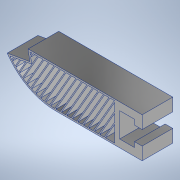
# Autodesk Inventor part: Finray_9_Kerbe_10deg_30deg20inf_PLA
Saved by Autodesk Inventor 2022 (Build 260153000, 153)
## iProperties
Created: 2022-02-28
Part Number: Finray_9_Kerbe_10deg_30deg20inf_PLA
Material: Generic
Document SubType Name: Modeling
Designer: richa
Density: 1 g/cm^3
Appearance: Aluminum - Flat
Author: richa
Autodesk Inventor part; units mm, degrees
ref_plane "YZ Plane" through (0, 0, 0) normal (1, 0, 0) x (0, 1, 0)
ref_plane "XZ Plane" through (0, 0, 0) normal (0, 1, 0) x (-1, 0, 0)
ref_plane "XY Plane" through (0, 0, 0) normal (0, 0, 1) x (1, 0, 0)
sketch "Sketch5" plane through (0, 0, 0) normal (0, 0, 1) x (1, 0, 0)
  line L0 (52.8, -15.6) -> (52.8, -10.6)
  line L1 (52.8, -10.6) -> (49.8, -10.6)
  line L2 (49.8, -10.6) -> (49.8, -12.6)
  line L3 (44, -12.6) -> (44, -3)
  line L4 (49.8, -3) -> (49.8, -5)
  line L5 (49.8, -5) -> (52.8, -5)
  line L6 (52.8, -5) -> (52.8, 0)
  line L7 (52.8, 0) -> (7.8, 0)
  line L8 (44, -3) -> (49.8, -3)
  line L9 (44, -12.6) -> (49.8, -12.6)
  line L10 (52.8, -15.6) -> (7.8, -15.6)
  line L11 (7.8, -15.6) -> (0, -15.6)
  line L12 (0, -15.6) -> (0, 0)
  line L13 (0, 0) -> (7.8, 0)
  point P0 (7.8, 0)
  dimension "d41" = 5.8
  dimension "d48" = 44
  dimension "d50" = 3
  dimension "d63" = 45
  dimension "d71" = 0
  dimension "d87" = 5.6
  dimension "d88" = 9.6
  dimension "d97" = 15.6
  constraints: 28 end point, 8 perpendicular, 4 collinear, 3 parallel, 2 horizontal, 1 vertical
  measures "d41" distance between parallel lines of L2 L3
  measures "d48" distance from line of L3 L12.end
  measures "d50" distance of L4.end L5.end
  measures "d63" distance of L0.start L10.end
  measures "d71" distance from line of L12.end L7
  measures "d87" distance from line of L0.end L5
  measures "d88" distance of L3.start L3.end
  measures "d97" distance of L11.end L12.end
extrude "Extrusion2" add sketch "Sketch5" along normal blind 12
sketch "Sketch8" plane through (0, 0, 0) normal (0, 0, -1) x (-1, 0, 0)
  line L0 (-8.1687, 0) -> (-8.8633, -3.9392)
  line L1 (-7.8, 0) -> (-1.143, 0) construction
  line L2 (0, -5.5021) -> (-8.8633, -3.9392)
  line L3 (-7.8, 0) -> (-8.1687, 0)
  line L4 (0, 0) -> (0, -15.6) projected
  line L5 (-52.8, 0) -> (0, 0) projected
  line L6 (-7.8, 0) -> (0, 0)
  line L7 (0, 0) -> (0, -5.5021)
  dimension "d80" = 100
  dimension "d95" = 4
  dimension "d96" = 9
  constraints: 12 end point, 2 collinear, 2 perpendicular, 1 horizontal, 1 point on line
  measures "d80" angle of L0 L1
  measures "d95" distance of L0.start L0.end
  measures "d96" distance of L2.start L0.end
extrude "Extrusion5" cut sketch "Sketch8" against normal through all
fillet "Fillet2" radius 23 1 edges at (0, -15.6, 6)
shell "Shell1" thickness 0.62 removed faces 1 at (23.9679, -7.5131, 12)
sketch "Sketch13" plane through (0, 0, 12) normal (0, 0, 1) x (1, 0, 0)
  line L0 (19.0404, -15.6) -> (52.8, -15.6) projected
  line L1 (42.0526, -15.6) -> (42.0526, 0)
  line L2 (52.8, 0) -> (8.1687, 0) projected
  line L3 (52.8, 0) -> (8.1687, 0) projected
  line L4 (52.8, -5) -> (52.8, 0) projected
  line L5 (49.8, -5) -> (52.8, -5) projected
  line L6 (49.8, -3) -> (49.8, -5) projected
  line L7 (44, -3) -> (49.8, -3) projected
  line L8 (44, -12.6) -> (44, -3) projected
  line L9 (49.8, -12.6) -> (44, -12.6) projected
  line L10 (49.8, -10.6) -> (49.8, -12.6) projected
  line L11 (52.8, -10.6) -> (49.8, -10.6) projected
  line L12 (52.8, -15.6) -> (52.8, -10.6) projected
  line L13 (42.0526, 0) -> (52.8, 0)
  line L14 (52.8, -5) -> (52.8, 0) projected
  line L15 (52.8, -5) -> (52.8, 0)
  line L16 (52.8, 0) -> (52.8, -5)
  line L17 (44, -12.6) -> (44, -3) projected
  line L18 (44, -3) -> (44, -12.6)
  line L19 (49.8, -12.6) -> (44, -12.6) projected
  line L20 (44, -12.6) -> (49.8, -12.6)
  line L21 (43.38, -13.22) -> (50.42, -13.22) projected
  line L22 (52.8, -10.6) -> (52.8, -15.6)
  line L23 (52.8, -15.6) -> (42.0526, -15.6)
  line L24 (44, -3) -> (49.8, -3) projected
  line L25 (44, -3) -> (49.8, -3)
  line L26 (49.8, -3) -> (49.8, -5)
  line L27 (49.8, -5) -> (52.8, -5)
  line L28 (52.8, -10.6) -> (49.8, -10.6)
  line L29 (49.8, -10.6) -> (49.8, -12.6)
  point P0 (0, 0)
  dimension "d102" = 10.7474
  constraints: 26 end point, 10 collinear, 2 point on line, 2 vertical, 1 parallel
  measures "d102" distance between parallel lines of L4 L1
extrude "Extrusion7" add sketch "Sketch13" against normal blind 12
sketch "Sketch14" plane through (8.9076, -0.62, 0.62) normal (0, 0, 1) x (1, 0, 0)
  line L0 (33.145, -14.36) -> (33.145, 0) projected
  line L1 (33.145, 0) -> (0, 0) projected
  line L2 (0.6739, -3.8221) -> (0, 0) projected
  line L3 (-7.835, -5.3225) -> (0.6739, -3.8221) projected
  arc A0 (-7.835, -5.3225) -> (10.1328, -14.36) centre (10.1328, 8.02) ccw projected
  line L4 (10.1328, -14.36) -> (33.145, -14.36) projected
  point P0 (-8.9076, 0.62)
extrude "Extrusion8" cut sketch "Sketch14" against normal blind 12
sketch "Sketch15" plane through (0, 0, 12) normal (0, 0, 1) x (1, 0, 0)
  line L0 (42.0526, -0.62) -> (8.9076, -0.62) construction
  line L1 (19.0404, -14.98) -> (42.0526, -14.98) projected
  line L2 (46.3521, -0.43) -> (46.6811, -0.62)
  line L3 (46.6811, -0.62) -> (38.2807, -15.17)
  line L4 (38.2807, -15.17) -> (37.9516, -14.98)
  line L5 (37.9516, -14.98) -> (46.3521, -0.43)
  arc A0 (1.0726, -5.9425) -> (19.0404, -14.98) centre (19.0404, 7.4) ccw projected
  line L6 (42.0526, -0.62) -> (42.0526, -14.98) projected
  line L7 (1.0726, -5.9425) -> (9.5815, -4.4421) projected
  arc A1 (0, -5.5021) -> (19.0404, -15.6) centre (19.0404, 7.4) ccw projected
  line L8 (42.0526, -14.98) -> (19.0404, -14.98) projected
  line L9 (8.9076, -0.62) -> (42.0526, -0.62) projected
  line L10 (42.3811, -0.62) -> (34.0904, -14.98)
  line L11 (41.9424, -0.62) -> (33.6516, -14.98)
  line L12 (33.7811, -0.62) -> (25.4904, -14.98)
  line L13 (33.3424, -0.62) -> (25.0516, -14.98)
  line L14 (29.4811, -0.62) -> (21.1904, -14.98)
  line L15 (29.0424, -0.62) -> (20.7516, -14.98)
  line L16 (25.1811, -0.62) -> (16.8904, -14.98)
  line L17 (24.7424, -0.62) -> (16.4516, -14.98)
  line L18 (20.8811, -0.62) -> (13.0602, -14.1662)
  line L19 (16.5811, -0.62) -> (9.5183, -12.8532)
  line L20 (16.1424, -0.62) -> (9.1748, -12.6882)
  line L21 (12.2811, -0.62) -> (6.2918, -10.9939)
  line L22 (11.8424, -0.62) -> (5.98, -10.7739)
  line L23 (7.9811, -0.62) -> (3.3805, -8.5885)
  line L24 (7.5424, -0.62) -> (3.102, -8.3109)
  line L25 (20.4424, -0.62) -> (12.6838, -14.0583)
  line L26 (38.0811, -0.62) -> (29.7904, -14.98)
  line L27 (37.6424, -0.62) -> (29.3516, -14.98)
  line L28 (42.0526, -14.98) -> (42.0526, -0.62) construction
  line L29 (42.0526, -0.62) -> (54.6606, -0.62) construction
  line L30 (44.5311, -0.62) -> (36.2404, -14.98)
  line L31 (44.0924, -0.62) -> (35.8016, -14.98)
  line L32 (40.2311, -0.62) -> (31.9404, -14.98)
  line L33 (39.7924, -0.62) -> (31.5016, -14.98)
  line L34 (35.9311, -0.62) -> (27.6404, -14.98)
  line L35 (35.4924, -0.62) -> (27.2016, -14.98)
  line L36 (31.6311, -0.62) -> (23.3404, -14.98)
  line L37 (31.1924, -0.62) -> (22.9016, -14.98)
  line L38 (27.3311, -0.62) -> (19.0404, -14.98)
  line L39 (26.8924, -0.62) -> (18.6041, -14.9757)
  line L40 (23.0311, -0.62) -> (14.9573, -14.6044)
  line L41 (22.5924, -0.62) -> (14.5629, -14.5275)
  line L42 (18.7311, -0.62) -> (11.2488, -13.5799)
  line L43 (18.2924, -0.62) -> (10.8891, -13.4428)
  line L44 (14.4311, -0.62) -> (7.8662, -11.9908)
  line L45 (13.9924, -0.62) -> (7.5386, -11.7983)
  line L46 (10.1311, -0.62) -> (4.7957, -9.8613)
  line L47 (9.6924, -0.62) -> (4.5002, -9.6131)
  line L48 (9.5815, -4.4421) -> (8.9076, -0.62) construction
  line L49 (8.9076, -0.62) -> (0, -0.62) construction
  line L50 (5.8311, -0.62) -> (2.0508, -7.1677)
  line L51 (5.3924, -0.62) -> (1.7905, -6.8586)
  point P0 (0, 0)
  point P1 (37.9516, -14.98)
  point P2 (5.3429, -5.1895)
  point P3 (4.8544, -5.2757)
  point P4 (38.3904, -14.98)
  point P5 (37.9516, -14.98)
  point P6 (33.6516, -14.98)
  point P7 (34.0904, -14.98)
  point P8 (29.3516, -14.98)
  point P9 (25.4904, -14.98)
  point P10 (20.7516, -14.98)
  point P11 (21.1904, -14.98)
  point P12 (19.1926, -14.98)
  point P13 (19.4987, -14.98)
  point P14 (42.0526, -1.1891)
  point P15 (42.0526, -6.9394)
  point P16 (16.533, -14.8391)
  point P17 (16.947, -14.8819)
  point P18 (42.0526, -4.153)
  point P19 (35.8016, -14.98)
  point P20 (42.0526, -4.913)
  point P21 (42.0526, -2.3376)
  point P22 (42.0526, -2.9287)
  point P23 (22.9016, -14.98)
  point P24 (2.4607, -5.6977)
  point P25 (2.9492, -5.6116)
  point P26 (42.0526, -8.6369)
  point P27 (42.0526, -7.8769)
  dimension "d105" = 0.38
  dimension "d130" = 120
  dimension "d132" = 120
  dimension "d133" = 0.38
  dimension "d135" = 0.38
  dimension "d136" = 0.38
  dimension "d137" = 0.38
  dimension "d138" = 0.38
  dimension "d139" = 0.38
  dimension "d140" = 0.38
  dimension "d141" = 0.38
  dimension "d143" = 0.38
  dimension "d152" = 120
  dimension "d155" = 4.3
  dimension "d156" = 4.3
  dimension "d157" = 4.3
  dimension "d158" = 4.3
  dimension "d159" = 4.3
  dimension "d160" = 4.3
  dimension "d161" = 4.3
  dimension "d162" = 4.3
  dimension "d164" = 4.3
  dimension "d165" = 0.38
  dimension "d166" = 2.15
  dimension "d167" = 2.15
  dimension "d168" = 0.38
  dimension "d169" = 0.38
  dimension "d170" = 2.15
  dimension "d171" = 0.38
  dimension "d172" = 2.15
  dimension "d173" = 0.38
  dimension "d174" = 2.15
  dimension "d176" = 0.38
  dimension "d177" = 2.15
  dimension "d178" = 0.38
  dimension "d180" = 2.15
  dimension "d181" = 0.38
  dimension "d182" = 2.15
  dimension "d184" = 0.38
  dimension "d185" = 2.15
  dimension "d186" = 2.15
  dimension "d187" = 0.38
  constraints: 88 end point, 38 parallel, 10 point on line, 2 horizontal, 1 perpendicular, 75 other
  measures "d105" distance between parallel lines of L3 L5
  measures "d130" angle of L0 L3
  measures "d132" angle of L0 L10
  measures "d133" distance between parallel lines of L10 L11
  measures "d135" distance between parallel lines of L13 L12
  measures "d136" distance between parallel lines of L15 L14
  measures "d137" distance between parallel lines of L17 L16
  measures "d138" distance between parallel lines of L25 L18
  measures "d139" distance between parallel lines of L20 L19
  measures "d140" distance between parallel lines of L22 L21
  measures "d141" distance between parallel lines of L24 L23
  measures "d143" distance between parallel lines of L26 L27
  measures "d152" angle of L0 L12
  measures "d155" distance of L10.start L2.end
  measures "d156" distance of L26.start L10.start
  measures "d157" distance of L12.start L26.start
  measures "d158" distance of L14.start L12.start
  measures "d159" distance of L16.start L14.start
  measures "d160" distance of L18.start L16.start
  measures "d161" distance of L19.start L18.start
  measures "d162" distance of L21.start L19.start
  measures "d164" distance of L23.start L21.start
  measures "d165" distance between parallel lines of L30 L31
  measures "d166" distance of L2.end L30.start
  measures "d167" distance of L32.start L10.start
  measures "d168" distance between parallel lines of L32 L33
  measures "d169" distance between parallel lines of L34 L35
  measures "d170" distance of L26.start L34.start
  measures "d171" distance between parallel lines of L37 L36
  measures "d172" distance of L36.start L12.start
  measures "d173" distance between parallel lines of L38 L39
  measures "d174" distance of L38.start L14.start
  measures "d176" distance between parallel lines of L40 L41
  measures "d177" distance of L16.start L40.start
  measures "d178" distance between parallel lines of L42 L43
  measures "d180" distance of L18.start L42.start
  measures "d181" distance between parallel lines of L45 L44
  measures "d182" distance of L19.start L44.start
  measures "d184" distance between parallel lines of L46 L47
  measures "d185" distance of L21.start L46.start
  measures "d186" distance of L23.start L50.start
  measures "d187" distance between parallel lines of L50 L51
extrude "Extrusion9" add sketch "Sketch15" against normal blind 12 contours A0 L39 L9 L38 | L15 L9 L14 L1 | A0 L17 L9 L16 | L37 L9 L36 L1 | A0 L41 L9 L40 | L13 L9 L12 L1 | A0 L25 L9 L18 | L35 L9 L34 L1 | A0 L43 L9 L42 | L27 L9 L26 L1 | A0 L20 L9 L19 | L33 L9 L32 L1 | A0 L45 L9 L44 | L11 L9 L6 L10 L1 | A0 L22 L9 L21 | L31 L6 L30 L1 | A0 L47 L7 L46 | L5 L6 L3 L1 | L1 L3 L4 | L7 L47 L9 L46 | L5 L2 L3 L6 | A0 L24 L7 L23 | A0 L51 L7 L50
sketch "Sketch16" plane through (0, 0, 12) normal (0, 0, 1) x (1, 0, 0)
  line L0 (49.8, -3) -> (49.8, -5) projected
  line L1 (44, -12.6) -> (49.8, -12.6)
  line L2 (49.8, -12.6) -> (49.8, -3)
  line L3 (49.8, -3) -> (44, -3)
  line L4 (44, -3) -> (44, -12.6)
  point P0 (0, 0)
  constraints: 8 end point, 2 parallel, 1 horizontal, 1 perpendicular
extrude "Extrusion10" cut sketch "Sketch16" against normal blind 12
sketch "Sketch17" plane through (0, 0, 12) normal (0, 0, 1) x (1, 0, 0)
  arc A0 (0, -5.5021) -> (19.0404, -15.6) centre (19.0404, 7.4) ccw projected
  line L0 (0, -5.5021) -> (8.8633, -3.9392)
  line L1 (52.8, 0) -> (8.1687, 0) projected
  line L2 (9.5815, -4.4421) -> (5.3429, -5.1895) projected
  line L3 (8.1687, 0) -> (8.8633, -3.9392)
  line L4 (7.6528, -4.1527) -> (0, -5.5021) projected
  line L5 (0, -5.5021) -> (8.1687, 0)
  point P0 (0, 0)
  point P1 (8.3884, -4.023)
  dimension "d190" = 4
  constraints: 6 end point, 1 perpendicular
  measures "d190" distance of L1.end L0.end
extrude "Extrusion11" cut sketch "Sketch17" against normal blind 12
equation "\"l1\" = 8"
equation "\"d1\" = 0.38"
body "Solid2"
